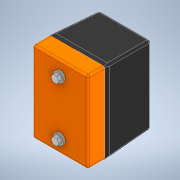
# Autodesk Inventor part: SuperBAndrena
Saved by Autodesk Inventor 2021 (Build 250183000, 183)
## iProperties
Created: 2020-10-24
Part Number: SuperBAndrena
Material: Generic
Document SubType Name: Modeling
Designer: lgnds
Density: 1 g/cm^3
Appearance: Default
Author: lgnds
Autodesk Inventor part; units mm, degrees
ref_plane "YZ Plane" through (0, 0, 0) normal (1, 0, 0) x (0, 1, 0)
ref_plane "XZ Plane" through (0, 0, 0) normal (0, 1, 0) x (-1, 0, 0)
ref_plane "XY Plane" through (0, 0, 0) normal (0, 0, 1) x (1, 0, 0)
sketch "Sketch1" plane through (0, 0, 0) normal (0, 0, 1) x (1, 0, 0)
  line L0 (-41, -60) -> (41, -60)
  line L1 (41, -60) -> (41, 60)
  line L2 (41, 60) -> (-41, 60)
  line L3 (-41, 60) -> (-41, -60)
  line L4 (-41, -60) -> (41, 60) construction
  line L5 (41, -60) -> (-41, 60) construction
  point P0 (0, 0)
  dimension "d0" = 120
  dimension "d1" = 82
  constraints: 12 end point, 2 midpoint, 2 parallel, 1 horizontal, 1 perpendicular
  measures "d0" distance of L2.end L0.start
  measures "d1" distance of L1.end L2.end
extrude "Extrusion1" add sketch "Sketch1" along normal blind 96
sketch "Sketch2" plane through (0, 0, 96) normal (0, 0, 1) x (1, 0, 0)
  line L0 (41, -60) -> (41, 60) projected
  line L1 (41, 60) -> (-41, 60) projected
  line L2 (-41, 60) -> (-41, -60) projected
  line L3 (-41, -60) -> (41, -60) projected
  point P0 (0, 0)
extrude "Extrusion2" cut sketch "Sketch2" against normal blind 25
sketch "Sketch3" plane through (0, 0, 71) normal (0, 0, 1) x (1, 0, 0)
  line L0 (-41, 60) -> (41, 60) projected
  line L1 (-41, -60) -> (-41, 60) projected
  line L2 (41, -60) -> (-41, -60) projected
  line L3 (41, 60) -> (41, -60) projected
  point P0 (0, 0)
extrude "Extrusion3" add sketch "Sketch3" along normal blind 25 separate body
chamfer "Chamfer1" distance 64.5 angle 2.5 1 edges at (41, 0, 0) measured on face at (41, 0, 0.5)
chamfer "Chamfer2" distance 64.5 angle 2.5 1 edges at (-1.4081, -60, 0) measured on face at (-1.4081, -60, 0.5)
chamfer "Chamfer3" distance 64.5 angle 2.5 1 edges at (-41, 1.4081, 0) measured on face at (-41, 1.4081, 0.5)
chamfer "Chamfer4" distance 64.5 angle 2.5 1 edges at (0, 60, 0) measured on face at (0, 60, 0.5)
sketch "Sketch4" plane through (0, 0, 96) normal (0, 0, 1) x (1, 0, 0)
  line L0 (-57.4, 0) -> (57.4, 0) projected
  line L1 (0, -84) -> (0, 84) projected
  circle A0 centre (0, -40) radius 7.5
  line L2 (-41, -60) -> (41, -60) projected
  point P0 (0, 0)
  dimension "d20" = 15
  dimension "d21" = 20
  constraints: 1 centre point, 1 point on line
  measures "d20" diameter of A0
  measures "d21" distance from line of L2 A0.centre
extrude "Extrusion4" add sketch "Sketch4" along normal blind 8 separate body
mirror "Mirror1" about plane through (0, 0, 0) normal (0, 1, 0) of "Extrusion4" bodies 3
fillet "Fillet1" radius 3 16 edges at (-39.5919, 58.5919, 32.25) (-39.5919, -58.5919, 32.25) (39.5919, -58.5919, 32.25) (39.5919, 58.5919, 32.25) (-38.1839, 0, 0) (0, 57.1839, 0) (38.1839, 0, 0) (0, -57.1839, 0) (-41, 60, 83.5) (-41, -60, 83.5) (41, -60, 83.5) (41, 60, 83.5) (41, 0, 96) (0, -60, 96) (-41, 0, 96) (0, 60, 96)
sketch "Sketch5" plane through (0, 40, 104) normal (0, 0, 1) x (1, 0, 0)
  circle A0 centre (0, 0) radius 7.5 projected
  circle A1 centre (0, -80) radius 7.5 projected
  circle A2 centre (0, 0) radius 7.5 projected
  line L0 (2.8868, 5) -> (5.7735, 0)
  line L1 (5.7735, 0) -> (2.8868, -5)
  line L2 (2.8868, -5) -> (-2.8868, -5)
  line L3 (-2.8868, -5) -> (-5.7735, 0)
  line L4 (-5.7735, 0) -> (-2.8868, 5)
  line L5 (-2.8868, 5) -> (2.8868, 5)
  circle A3 centre (0, -80) radius 7.5 projected
  line L6 (2.8868, -75) -> (5.7735, -80)
  line L7 (5.7735, -80) -> (2.8868, -85)
  line L8 (2.8868, -85) -> (-2.8868, -85)
  line L9 (-2.8868, -85) -> (-5.7735, -80)
  line L10 (-5.7735, -80) -> (-2.8868, -75)
  line L11 (-2.8868, -75) -> (2.8868, -75)
  point P0 (0, -40)
  dimension "d25" = 10
  dimension "d26" = 10
  constraints: 24 end point, 2 coincident, 2 horizontal, 26 other
  measures "d25" distance between parallel lines of L3 L0
  measures "d26" distance between parallel lines of L9 L6
extrude "Extrusion5" cut sketch "Sketch5" against normal blind 5 bodies 3
equation "\"d26\" = d25"
body "Solid1"
body "Solid2"
body "Solid3"
